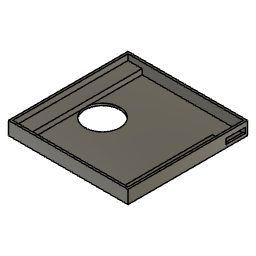
Matrix Boden (Autodesk Fusion 360 design; units mm, degrees)
Autodesk Fusion 360 part; units mm, degrees
box "Grundkörper Quader1" add length 65.5 width 65.5 height 6 placed x (0, 1, 0) y (-1, 0, 0) z (0, 0, 1) at (65.5, 0, 0) makes body 1
extrude "Extrusion2" add 1 faces at (43.6667, 0, 2) along direction (0, -1, 0) blind 2.4 on bodies 1 bodies 1
extrude "Extrusion3" add 1 faces at (65.5, 42.8667, 2) along direction (1, 0, 0) blind 2.4 on bodies 1 bodies 1
shell "Schale2" thickness 1.2 removed faces 1 at (45.2667, 20.2333, 6) on bodies 1
extrude "Extrusion4" add 1 faces at (67.5, 20.6333, 6) along direction (0, 0, 1) blind 1.5 on bodies 1 bodies 1
box "Grundkörper Quader5" add length 3 width 11 height 5 placed x (0, 0, 1) y (0, -1, 0) z (1, 0, 0) at (67.9, 62.3074, 3.5277) separate body makes body 2
move_body "Verschieben2" bodies 2 to x (1, 0, 0) y (0, 1, 0) z (0, 0, 1) at (0, 0, -2.328)
move_body "Verschieben3" bodies 2 to x (1, 0, 0) y (0, 1, 0) z (0, 0, 1) at (0, 2, 0)
move_body "Verschieben4" bodies 2 to x (1, 0, 0) y (0, 1, 0) z (0, 0, 1) at (-2, 0, 0)
move_body "Verschieben5" bodies 2 to x (1, 0, 0) y (0, 1, 0) z (0, 0, 1) at (0.0754, 0.0388, 0.5)
move_body "Verschieben6" bodies 2 to x (1, 0, 0) y (0, 1, 0) z (0, 0, 1) at (0, -0.0461, 0)
combine "Kombinieren2" operation cut target body 1 tool bodies 2
box "Grundkörper Quader6" add length 65.5 width 5 height 3 placed x (0, 1, 0) y (-1, 0, 0) z (0, 0, 1) at (6.2, -1.2, 1.2) separate body makes body 3
box "Grundkörper Quader7" add length 53 width 5 height 3 placed x (0, 1, 0) y (-1, 0, 0) z (0, 0, 1) at (66.7, -1.2, 1.2) separate body makes body 4
combine "Kombinieren3" operation add target body 1 tool bodies 4
combine "Kombinieren4" operation add target body 1 tool bodies 3
extrude "Extrusion5" add 1 faces at (6.2, 42.4667, 2.2) along direction (1, 0, 0) blind 3 on bodies 1 bodies 1
cylinder "Grundkörper Zylinder1" cut diameter 20 height -2 placed x (1, 0, 0) y (0, 1, 0) z (0, 0, 1) at (19, 32, 1.2) bodies 1
named bodies: "Rahmen", "Auflage1", "Auflage2"
